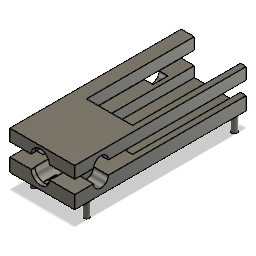
Atari 7800 AV MKII v5 (Autodesk Fusion 360 design; units mm, degrees)
Autodesk Fusion 360 part; units mm, degrees
note: some values were not read from the file. Chosen so that the rebuilt part matches the saved one: which face or edge a step refers to; which pieces of a blend or face edit are solid. Set by a fixed rule: which sketch regions a step uses.
sketch "Sketch1" plane through (0, 0, 0) normal (0, 1, 0) x (1, 0, 0)
  line L0 (0, 0) -> (22, 0)
  line L1 (22, 0) -> (22, -52.5)
  line L2 (22, -52.5) -> (0, -52.5)
  line L3 (0, -52.5) -> (0, 0)
  dimension "d1" = 22
  dimension "d2" = 52.5
  constraint horizontal L0
  constraint vertical L1
  constraint horizontal L2
  constraint vertical L3
  constraint coincident L0.start L3.end
  measures "d1" distance of L0.start L0.end
  measures "d2" distance of L0.start L2.end
extrude "Extrude1" add sketch "Sketch1" along normal blind 2 makes body 1
sketch "Sketch2" plane through (0, 0, 0) normal (0, -1, 0) x (1, 0, 0)
  line L0 (22, 52.5) -> (0, 52.5)
  line L1 (0, 52.5) -> (0, 0)
  line L2 (0, 0) -> (22, 0)
  line L3 (22, 0) -> (22, 52.5)
  line L4 (0, 0) -> (1.35, 0)
  circle A0 centre (1.35, 1) radius 1
  dimension "d5" = 1.35
  dimension "d6" = 2
  constraint coincident L1.end L2.start
  constraint coincident L4.end A0
  measures "d5" distance of L1.end L4.end
  measures "d6" diameter of A0
extrude "Extrude2" add sketch "Sketch2" along normal blind 5 contours A0 bodies 1
sketch "Sketch3" plane through (0, 0, 0) normal (0, 1, 0) x (1, 0, 0)
  line L0 (1.35, 0) -> (17.05, 0)
  circle A0 centre (17.05, -1) radius 1
  point P0 (1.35, 0)
  dimension "d9" = 15.7
  dimension "d10" = 2
  constraint coincident P0 L0.start
  constraint coincident L0.end A0
  measures "d9" distance of P0 L0.end
  measures "d10" diameter of A0
extrude "Extrude3" add sketch "Sketch3" against normal blind 5 bodies 1
sketch "Sketch4" plane through (0, 0, 0) normal (0, 1, 0) x (1, 0, 0)
  line L0 (1.35, -1.9999) -> (1.35, -2.1921)
  line L1 (1.35, -2.1921) -> (1.35, -50.1921)
  circle A0 centre (1.35, -51.1921) radius 1
  point P0 (1.35, 0)
  dimension "d13" = 48
  dimension "d14" = 2
  constraint coincident L1.end A0
  measures "d13" distance of L0.end L1.end
  measures "d14" diameter of A0
extrude "Extrude4" add sketch "Sketch4" against normal blind 5 bodies 1
sketch "Sketch5" plane through (0, 0, 0) normal (0, -1, 0) x (1, 0, 0)
  circle A0 centre (1.35, 51.1921) radius 1
  line L0 (22, 52.5) -> (0, 52.5)
  line L1 (0, 52.5) -> (0, 0)
  line L2 (0, 0) -> (1.35, 0)
  circle A1 centre (1.35, 1) radius 1
  line L3 (1.35, 0) -> (17.05, 0)
  circle A2 centre (17.05, 1) radius 1
  line L4 (17.05, 0) -> (22, 0)
  line L5 (22, 0) -> (22, 52.5)
  line L6 (1.35, 51.1921) -> (1.35, 52.1921)
  line L7 (1.35, 52.1921) -> (17.05, 52.1921)
  circle A3 centre (17.05, 51.1921) radius 1
  dimension "d17" = 15.7
  dimension "d18" = 2
  constraint coincident A0.centre L6.start
  constraint vertical L6
  constraint coincident L7.end A3
  measures "d17" distance of L6.end L7.end
  measures "d18" diameter of A3
extrude "Extrude5" add sketch "Sketch5" along normal blind 5 contours A3 bodies 1
sketch "Sketch6" plane through (0, 0, 52.5) normal (0, 0, 1) x (1, 0, 0)
  line L0 (0, 0) -> (22, 0)
  line L1 (22, 0) -> (22, 2)
  line L2 (22, 2) -> (0, 2)
  line L3 (0, 2) -> (0, 0)
  line L4 (0, 2) -> (13.35, 2)
  line L5 (13.35, 2) -> (13.35, 9)
  circle A0 centre (13.35, 9) radius 3
  dimension "d21" = 13.35
  dimension "d22" = 7
  dimension "d23" = 6
  constraint coincident L2.end L3.start
  constraint coincident L5.end A0.centre
  measures "d21" distance of L2.end L4.end
  measures "d22" distance of L4.end L5.end
  measures "d23" diameter of A0
extrude "Extrude6" add sketch "Sketch6" along normal blind 3 separate body contours A0 makes body 2
sketch "Sketch7" plane through (0, 0, 52.5) normal (0, 0, -1) x (-1, 0, 0)
  circle A0 centre (-13.35, 9) radius 3
  circle A1 centre (-13.35, 9) radius 3.225
  dimension "d26" = 6.45
  constraint concentric A0 A1
  measures "d26" diameter of A1
extrude "Extrude7" add sketch "Sketch7" along normal blind 14.7 contours A0 | A1 bodies 2
sketch "Sketch8" plane through (0, 0, 37.8) normal (0, 0, -1) x (-1, 0, 0)
  circle A0 centre (-13.35, 9) radius 3.225
  circle A1 centre (-13.35, 9) radius 2.725
  dimension "d29" = 5.45
  constraint concentric A0 A1
  measures "d29" diameter of A1
extrude "Extrude8" add sketch "Sketch8" along normal blind 2 and the other way blind -0.5 separate body makes body 3
sketch "Sketch9" plane through (0, 0, 55.5) normal (0, 0, 1) x (1, 0, 0)
  circle A0 centre (13.35, 9) radius 3
  circle A1 centre (13.35, 9) radius 3.075
  circle A2 centre (13.35, 9) radius 3.225
  circle A3 centre (13.35, 9) radius 3.225
  dimension "d34" = 6.15
  constraint concentric A0 A1
  constraint concentric A1 A2
  measures "d34" diameter of A1
extrude "Extrude9" add sketch "Sketch9" along normal blind -2.8 and the other way blind 0.2 separate body contours A2 A3 makes body 4
extrude "Extrude10" add 1 faces at (10.3138, 8.7044, 37.3) along direction (0, 0, 1) blind 0.3 on bodies 3 bodies 3
sketch "Sketch10" plane through (0, 2, 0) normal (0, 1, 0) x (-1, 0, 0)
  line L0 (0, 52.5) -> (-22, 52.5)
  line L1 (-22, 52.5) -> (-22, 0)
  line L2 (-22, 0) -> (0, 0)
  line L3 (0, 0) -> (0, 52.5)
  line L4 (-16.575, 35.8) -> (-10.125, 35.8)
  line L5 (-10.2258, 35.8) -> (1.5, 35.8)
  line L6 (-16.075, 37.6) -> (-26, 37.6)
  line L7 (-22, 37.6) -> (0, 37.6)
  line L8 (0, 37.6) -> (0, 35.8)
  line L9 (0, 35.8) -> (-22, 35.8)
  line L10 (-22, 35.8) -> (-22, 37.6)
  point P0 (-16.075, 37.6)
  constraint coincident L4 L5.start
  constraint perpendicular L3 L5
  constraint coincident P0 L6.start
  constraint parallel L4 L6
  constraint horizontal L7
  constraint vertical L8
  constraint horizontal L9
  constraint vertical L10
  constraint coincident L5 L8.end
  constraint coincident L3 L8.end
  constraint coincident L6 L7.start
  constraint coincident L1 L7.start
extrude "Extrude11" add sketch "Sketch10" along normal blind 4 contours L1 L3 L4 L5 L6 L7 L8 L9 L10 bodies 3 1
sketch "Sketch11" plane through (0, 0, 35.8) normal (0, 0, -1) x (-1, 0, 0)
  arc A0 (-12.1665, 6) -> (-14.5335, 6) centre (-13.35, 9) ccw
  line L0 (-14.5335, 6) -> (-22, 6)
  line L1 (-22, 6) -> (-22, 2)
  line L2 (-22, 2) -> (0, 2)
  line L3 (0, 2) -> (0, 6)
  line L4 (0, 6) -> (-12.1665, 6)
  circle A1 centre (-13.35, 9) radius 2.725
  line L5 (-13.35, 9) -> (-22, 9)
  line L6 (-22, 9) -> (-22, 6)
  line L7 (-13.35, 9) -> (0, 9)
  line L8 (0, 9) -> (0, 6)
  constraint coincident A0.centre A1.centre
  constraint horizontal L5
  constraint coincident L0.end L1.start
  constraint perpendicular L5 L6
  constraint perpendicular L6 L7
  constraint coincident L3.end L4.start
  constraint perpendicular L4 L8
extrude "Extrude12" add sketch "Sketch11" against normal blind 1.8 contours A0 L4 L7 L8 | A0 L0 L5 L6 bodies 3
sketch "Sketch12" plane through (0, 0, 37.6) normal (0, 0, 1) x (1, 0, 0)
  arc A0 (16.575, 9) -> (10.125, 9) centre (13.35, 9) ccw
  line L0 (10.125, 9) -> (0, 9)
  line L1 (0, 9) -> (0, 2)
  line L2 (0, 2) -> (22, 2)
  line L3 (22, 2) -> (22, 9)
  line L4 (22, 9) -> (16.575, 9)
  circle A1 centre (13.35, 9) radius 2.725
  circle A2 centre (13.35, 9) radius 3.25
  dimension "d45" = 6.5
  constraint concentric A0 A2
  measures "d45" diameter of A2
extrude "Extrude13" add sketch "Sketch12" along normal blind 14.5 contours L0 L1 L2 L3 L4 A2 bodies 3
extrude "Extrude14" add 1 faces at (14.6667, 0.6667, 52.5) along direction (0, 0, 1) blind 1 on bodies 3 bodies 3
extrude "Extrude15" add 1 faces at (7.3333, 2, 53.0333) along direction (0, 1, 0) blind 3.8 on bodies 3 bodies 3 4
extrude "Extrude16" add 1 faces at (3.3772, 7.7827, 52.1) along direction (0, 0, 1) blind 1.4 on bodies 3 bodies 3
extrude "Extrude17" add 1 faces at (20.1581, 7.635, 52.1) along direction (0, 0, 1) blind 1.4 on bodies 3 bodies 3
sketch "Sketch13" plane through (22, 0, 0) normal (1, 0, 0) x (0, 0, -1)
  line L0 (-35.8, 2) -> (-35.8, 9)
  line L1 (-35.8, 9) -> (-53.5, 9)
  line L2 (-53.5, 9) -> (-53.5, 0)
  line L3 (-53.5, 0) -> (0, 0)
  line L4 (0, 0) -> (0, 2)
  line L5 (0, 2) -> (-35.8, 2)
  line L6 (-35.8, 9) -> (-56, 9)
  line L7 (-56, 9) -> (-56, 13)
  line L8 (-56, 13) -> (-35.8, 13)
  line L9 (-35.8, 13) -> (-35.8, 9)
  constraint horizontal L6
  constraint vertical L7
  constraint horizontal L8
  constraint vertical L9
  constraint coincident L0.end L1.start
extrude "Extrude18" cut sketch "Sketch13" against normal blind 21 contours L1 L6 L7 L8 L9 bodies 3
extrude "Extrude19" cut 1 faces at (13.2164, 5.8, 52.3) along direction (0, -1, 0) blind 0.1 on bodies 3 bodies 3
extrude "Extrude20" add 1 faces at (12.9492, 5.7667, 52.9667) along direction (1, 0, 0) blind 1.3 on bodies 3 bodies 3
extrude "Extrude21" add 1 faces at (12.9492, 5.7667, 52.9667) along direction (-1, 0, 0) blind 0.69 on bodies 3 bodies 3
extrude "Extrude22" add 1 faces at (12.8935, 5.8, 53.2333) along direction (0, 1, 0) blind 0.05 on bodies 3 bodies 3
extrude "Extrude23" add 1 faces at (13.8065, 5.8, 53.2333) along direction (0, 1, 0) blind 0.06 on bodies 3 bodies 3
move_face "OffsetFaces1" offset 0.6 1 faces at (14.2695, 5.9089, 53.8333) on bodies 3
extrude "Extrude24" cut 1 faces at (16.9108, 8.81, 55.3) along direction (0, 0, -1) blind 1.8 on bodies 3 bodies 3
extrude "Extrude25" add 1 faces at (3.5265, 5.5553, 53.5) along direction (0, 0, 1) blind 0.5 on bodies 3 bodies 3
extrude "Extrude26" add 1 faces at (7.3333, 2, 11.9333) along direction (0, 1, 0) blind 7 on bodies 3 bodies 3
extrude "Extrude27" cut 1 faces at (12.7837, 8.2898, 35.8) along direction (0, 0, -1) blind 36 on bodies 3 bodies 3
sketch "Sketch14" plane through (0, 9, 0) normal (0, 1, 0) x (-1, 0, 0)
  line L0 (-16.075, 0) -> (-16.075, 37.6)
  line L1 (-16.075, 37.6) -> (-16.6, 37.6)
  line L2 (-16.6, 37.6) -> (-16.6, 52.7)
  line L3 (-16.6, 52.7) -> (-16.425, 52.7)
  line L4 (-16.425, 52.7) -> (-16.425, 54)
  line L5 (-16.425, 54) -> (-22, 54)
  line L6 (-22, 54) -> (-22, 0)
  line L7 (-22, 0) -> (-16.075, 0)
  line L8 (-20, 0) -> (-4.4651, 0)
  line L9 (-4.4651, 0) -> (-4.4651, 32.4674)
  line L10 (-4.4651, 32.4674) -> (-20, 32.4674)
  line L11 (-20, 32.4674) -> (-20, 0)
  constraint horizontal L8
  constraint vertical L9
  constraint horizontal L10
  constraint vertical L11
  constraint coincident L7 L8.start
extrude "Extrude28" cut sketch "Sketch14" against normal blind 4 contours L0 L7 L8 L10 L11 | L0 L8 L9 L10 bodies 3
sketch "Sketch15" plane through (0, 0, 54) normal (0, 0, 1) x (1, 0, 0)
  line L0 (10.275, 9) -> (0, 9)
  line L1 (0, 9) -> (0, 0)
  line L2 (0, 0) -> (22, 0)
  line L3 (22, 0) -> (22, 9)
  line L4 (22, 9) -> (16.425, 9)
  arc A0 (10.275, 9) -> (16.425, 9) centre (13.35, 9) ccw
  line L5 (0, 9) -> (22, 9)
  line L6 (22, 9) -> (22, 13)
  line L7 (22, 13) -> (0, 13)
  line L8 (0, 13) -> (0, 9)
  dimension "d79" = 4
  constraint horizontal L5
  constraint vertical L6
  constraint horizontal L7
  constraint vertical L8
  constraint coincident L0.end L1.start
  measures "d79" distance of L0.end L7.end
extrude "Extrude29" add sketch "Sketch15" against normal blind 54 separate body contours L0 L4 L5 L6 L7 L8 makes body 5
sketch "Sketch16" plane through (0, 0, 54) normal (0, 0, 1) x (1, 0, 0)
  line L0 (10.275, 9) -> (0, 9)
  line L1 (0, 9) -> (0, 0)
  line L2 (0, 0) -> (22, 0)
  line L3 (22, 0) -> (22, 9)
  line L4 (22, 9) -> (16.425, 9)
  arc A0 (10.275, 9) -> (16.425, 9) centre (13.35, 9) ccw
  circle A1 centre (13.35, 9) radius 3.075
  constraint concentric A0 A1
extrude "Extrude30" cut sketch "Sketch16" against normal blind 16 contours A0 A1 bodies 5
sketch "Sketch17" plane through (0, 0, 37.6) normal (0, 0, 1) x (1, 0, 0)
  line L0 (10.625, 9) -> (10.1, 9)
  arc A0 (10.1, 9) -> (16.6, 9) centre (13.35, 9) ccw
  line L1 (16.6, 9) -> (16.075, 9)
  arc A1 (10.625, 9) -> (16.075, 9) centre (13.35, 9) ccw
  circle A2 centre (13.35, 9) radius 3.25
  constraint concentric A0 A2
extrude "Extrude31" cut sketch "Sketch17" along normal blind 15.1 bodies 5
sketch "Sketch18" plane through (0, 0, 37.6) normal (0, 0, 1) x (1, 0, 0)
  line L0 (10.625, 9) -> (10.1, 9)
  arc A0 (10.1, 9) -> (16.6, 9) centre (13.35, 9) ccw
  line L1 (16.6, 9) -> (16.075, 9)
  arc A1 (10.625, 9) -> (16.075, 9) centre (13.35, 9) ccw
  circle A2 centre (13.35, 9) radius 2.725
  constraint concentric A0 A2
extrude "Extrude32" cut sketch "Sketch18" against normal blind 40 contours A1 A2 bodies 5
extrude "Extrude33" cut 1 faces at (12.205, 5, 21.6449) along direction (0, 1, 0) blind 10 on bodies 3 bodies 5
extrude "Extrude34" cut 1 faces at (1.6126, -5, 51.6617) along direction (0, 1, 0) blind 5 on bodies 3 bodies 3
extrude "Extrude35" cut 1 faces at (16.7497, -5, 51.3367) along direction (0, 1, 0) blind 5 on bodies 3 bodies 3
extrude "Extrude36" cut 1 faces at (16.476, -5, 0.7236) along direction (0, 1, 0) blind 5 on bodies 3 bodies 3
sketch "Sketch19" plane through (0, 0, 0) normal (0, -1, 0) x (1, 0, 0)
  line L0 (0, 54) -> (0, 0)
  line L1 (0, 0) -> (1.35, 0)
  circle A0 centre (1.35, 1) radius 1
  line L2 (1.35, 0) -> (22, 0)
  line L3 (22, 0) -> (22, 54)
  line L4 (22, 54) -> (0, 54)
  line L5 (0, 54) -> (0, 53)
  circle A1 centre (1, 53) radius 1
  dimension "d96" = 1
  dimension "d97" = 2
  constraint coincident L0.start L4.end
  constraint coincident L5.end A1
  measures "d96" distance of L0.start L5.end
  measures "d97" diameter of A1
extrude "Extrude37" add sketch "Sketch19" along normal blind 5 contours A1 bodies 3
sketch "Sketch20" plane through (0, 0, 0) normal (0, -1, 0) x (1, 0, 0)
  arc A0 (0, 53) -> (1, 54) centre (1, 53) ccw
  line L0 (0, 53) -> (0, 0)
  line L1 (0, 0) -> (1.35, 0)
  circle A1 centre (1.35, 1) radius 1
  line L2 (1.35, 0) -> (22, 0)
  line L3 (22, 0) -> (22, 54)
  line L4 (22, 54) -> (1, 54)
  line L5 (22, 54) -> (22, 53)
  circle A2 centre (21, 53) radius 1
  dimension "d100" = 1
  dimension "d101" = 2
  constraint coincident L3.end L4.start
  constraint coincident L3 L5.end
  constraint perpendicular L4 L5
  constraint coincident L5.end A2
  measures "d100" distance of L3.end L5.end
  measures "d101" diameter of A2
extrude "Extrude38" add sketch "Sketch20" along normal blind 5 contours A2 bodies 3
sketch "Sketch21" plane through (0, 0, 0) normal (0, -1, 0) x (1, 0, 0)
  arc A0 (21, 54) -> (22, 53) centre (21, 53) ccw
  line L0 (21, 54) -> (1, 54)
  arc A1 (0, 53) -> (1, 54) centre (1, 53) ccw
  line L1 (0, 53) -> (0, 0)
  line L2 (0, 0) -> (1.35, 0)
  circle A2 centre (1.35, 1) radius 1
  line L3 (1.35, 0) -> (22, 0)
  line L4 (22, 0) -> (22, 53)
  line L5 (22, 0) -> (21, 0)
  circle A3 centre (21, 1) radius 1
  dimension "d104" = 1
  dimension "d105" = 2
  constraint coincident L3.end L4.start
  constraint coincident L5.end A3
  measures "d104" distance of L3.end L5.end
  measures "d105" diameter of A3
extrude "Extrude39" add sketch "Sketch21" along normal blind 5 contours A3 bodies 3
sketch "Sketch22" plane through (4.4651, 0, 0) normal (1, 0, 0) x (0, 0, -1)
  line L0 (0, 9) -> (-32.4674, 9)
  line L1 (-32.4674, 9) -> (-32.4674, 5)
  line L2 (-32.4674, 5) -> (0, 5)
  line L3 (0, 5) -> (0, 9)
  line L4 (0, 5) -> (-5, 5)
  line L5 (-5, 5) -> (-5, 6)
  line L6 (-5, 6) -> (0, 6)
  line L7 (0, 6) -> (0, 5)
  line L8 (-5, 6) -> (-7.5, 6)
  line L9 (-7.5, 6) -> (-7.5, 5)
  line L10 (-7.5, 5) -> (-5, 5)
  line L11 (-5, 5) -> (-5, 6)
  line L12 (-7.5, 6) -> (-10, 6)
  line L13 (-10, 6) -> (-10, 5)
  line L14 (-10, 5) -> (-7.5, 5)
  line L15 (-7.5, 5) -> (-7.5, 6)
  line L16 (-10, 6) -> (-12.5, 6)
  line L17 (-12.5, 6) -> (-12.5, 5)
  line L18 (-12.5, 5) -> (-10, 5)
  line L19 (-10, 5) -> (-10, 6)
  line L20 (-12.5, 6) -> (-10, 6)
  line L21 (-10, 6) -> (-10, 9)
  line L22 (-10, 9) -> (-12.5, 9)
  line L23 (-12.5, 9) -> (-12.5, 6)
  line L24 (-7.5, 6) -> (-5, 6)
  line L25 (-5, 6) -> (-5, 9)
  line L26 (-5, 9) -> (-7.5, 9)
  line L27 (-7.5, 9) -> (-7.5, 6)
  line L28 (-12.5, 9) -> (-5, 9)
  line L29 (-5, 9) -> (-5, 8)
  line L30 (-5, 8) -> (-12.5, 8)
  line L31 (-12.5, 8) -> (-12.5, 9)
  dimension "d108" = 5
  dimension "d109" = 1
  dimension "d110" = 1
  dimension "d111" = 2.5
  dimension "d112" = 2.5
  dimension "d113" = 1
  dimension "d114" = 2.5
  dimension "d115" = 1
  constraint horizontal L4
  constraint vertical L5
  constraint horizontal L6
  constraint vertical L7
  constraint coincident L2.end L3.start
  constraint horizontal L8
  constraint vertical L9
  constraint horizontal L10
  constraint vertical L11
  constraint horizontal L12
  constraint vertical L13
  constraint horizontal L14
  constraint vertical L15
  constraint horizontal L16
  constraint vertical L17
  constraint horizontal L18
  constraint vertical L19
  constraint horizontal L20
  constraint vertical L21
  constraint horizontal L22
  constraint vertical L23
  constraint coincident L0 L21.end
  constraint horizontal L24
  constraint vertical L25
  constraint horizontal L26
  constraint vertical L27
  constraint coincident L0 L25.end
  constraint horizontal L28
  constraint vertical L29
  constraint horizontal L30
  constraint vertical L31
  constraint coincident L25 L29.end
  measures "d108" distance of L2.end L4.end
  measures "d109" distance of L2.end L6.end
  measures "d110" distance of L5.end L4.end
  measures "d111" distance of L5.end L8.end
  measures "d112" distance of L8.end L12.end
  measures "d113" distance of L8.end L9.end
  measures "d114" distance of L12.end L16.end
  measures "d115" distance of L12.end L13.end
extrude "Extrude40" add sketch "Sketch22" along normal blind 17 contours L0 L25 L26 L27 L28 L29 L30 | L0 L21 L22 L23 L28 L30 L31 bodies 3
extrude "Extrude41" cut 1 faces at (1.2554, -5, 53.3747) along direction (0, 1, 0) blind 5 on bodies 3 bodies 3
extrude "Extrude42" cut 1 faces at (1.0981, -5, 1.5651) along direction (0, 1, 0) blind 5 on bodies 3 bodies 3
extrude "Extrude43" cut 1 faces at (20.5597, -5, 0.788) along direction (0, 1, 0) blind 5 on bodies 3 bodies 3
sketch "Sketch23" plane through (0, 0, 0) normal (0, -1, 0) x (1, 0, 0)
  line L0 (21, 54) -> (0, 54)
  line L1 (0, 54) -> (0, 0)
  line L2 (0, 0) -> (22, 0)
  line L3 (22, 0) -> (22, 53)
  arc A0 (21, 54) -> (22, 53) centre (21, 53) ccw
  circle A1 centre (21, 3) radius 1
  circle A2 centre (3.35, 3) radius 1
  circle A3 centre (3.35, 53) radius 1
  dimension "d124" = 50
  dimension "d125" = 2
  dimension "d126" = 17.65
  dimension "d127" = 2
  dimension "d128" = 50
  dimension "d129" = 2
  measures "d124" distance of A0.centre A1.centre
  measures "d125" diameter of A1
  measures "d126" distance of A1.centre A2.centre
  measures "d127" diameter of A2
  measures "d128" distance of A2.centre A3.centre
  measures "d129" diameter of A3
extrude "Extrude44" add sketch "Sketch23" along normal blind 5 contours A3 | A1 | A2 bodies 3
move_face "MoveFace1" to x (1, 0, 0) y (0, 1, 0) z (0, 0, 1) at (-3, 0, 0) 11 faces at (13.2733, 5.926, 53.6667) (13.4267, 5.926, 53.2333) (13.2734, 5.7779, 52.7) (11.523, 6.3122, 42.6333) (16.4028, 8.7032, 37.6) (10.6385, 8.7287, 37) (10.6385, 8.7287, 34.6891) (12.7821, 5.7333, 52.5) (13.5393, 5.7, 52.3) (13.9179, 5.7333, 52.5) (13.792, 5.7519, 52.1) on bodies 3
move_face "MoveFace2" to x (1, 0, 0) y (0, 1, 0) z (0, 0, 1) at (-3, 0, 0) 5 faces at (11.3153, 11.3056, 53.5667) (16.596, 9.162, 42.6333) (16.4028, 9.2968, 37.6) (15.9907, 9.6724, 34.1783) (16.5181, 9.3142, 52.7) on bodies 5
sketch "Sketch24" plane through (0, 0, 0) normal (-1, 0, 0) x (0, 0, 1)
  line L0 (54, 9) -> (0, 9)
  line L1 (0, 9) -> (0, 0)
  line L2 (0, 0) -> (54, 0)
  line L3 (54, 0) -> (54, 9)
  circle A0 centre (10, 9) radius 2.5
  circle A1 centre (45.15, 9) radius 2.5
  line L4 (52.7, 9) -> (37.6, 9)
  point P0 (10, 9)
  dimension "d132" = 5
  dimension "d133" = 5
  constraint coincident P0 A0.centre
  constraint midpoint A1.centre L4
  measures "d132" diameter of A0
  measures "d133" diameter of A1
extrude "Extrude45" cut sketch "Sketch24" against normal blind 3 contours L0 A1 L4 | L0 A1 L4 | L0 A0 | L0 A0 bodies 3 5
sketch "Sketch25" plane through (22, 0, 0) normal (1, 0, 0) x (0, 0, -1)
  line L0 (0, 9) -> (-54, 9)
  line L1 (-54, 9) -> (-54, 0)
  line L2 (-54, 0) -> (-53, 0)
  line L3 (-53, 0) -> (-3, 0)
  line L4 (-3, 0) -> (0, 0)
  line L5 (0, 0) -> (0, 9)
  circle A0 centre (-45.15, 9) radius 2.5
  line L6 (-47.65, 9) -> (-42.65, 9)
  dimension "d136" = 5
  constraint midpoint A0.centre L6
  measures "d136" diameter of A0
extrude "Extrude46" cut sketch "Sketch25" against normal blind 5 contours L0 A0 L6 | L0 A0 L6 bodies 3 5
extrude "Extrude47" cut 2 faces at (3, 9.3616, 45.9008) (3, 8.3928, 44.3622) along direction (1, 0, 0) blind 2 on bodies 3 5 bodies 3 5
move_face "MoveFace3" to x (1, 0, 0) y (0, 1, 0) z (0, 0, 1) at (0, 0, 4) 11 faces at (18.7068, 5.5553, 54) (12.3847, 6.6944, 53.1333) (18.6667, 8.8754, 42.6531) (2, 8.8754, 47.6469) (4.3333, 8.8754, 47.6469) (5, 8.3928, 44.3622) (17, 8.3928, 45.9378) (10.4266, 5.7779, 52.7) (13.4028, 8.7032, 37.6) (7.6385, 8.7287, 35.8891) (17.6513, 7.3989, 32.4674) on bodies 3
extrude "Extrude48" add 1 faces at (9.6434, 8.6667, 12.5) along direction (0, 0, 1) blind 7 on bodies 3 bodies 3
extrude "Extrude49" cut 1 faces at (9.6434, 8.3333, 10) along direction (0, 0, 1) blind 7 on bodies 3 bodies 3
extrude "Extrude50" add 1 faces at (9.6434, 8.6667, 7.5) along direction (0, 0, 1) blind 5 on bodies 3 bodies 3
extrude "Extrude51" cut 1 faces at (9.6434, 8.6667, 5) along direction (0, 0, 1) blind 5 on bodies 3 bodies 3
move_face "MoveFace4" to x (1, 0, 0) y (0, 1, 0) z (0, 0, 1) at (0, 0, 4) 9 faces at (19.0961, 10.6355, 54) (1.6667, 9.2489, 42.6624) (17.5333, 9, 51.45) (8.3153, 11.3056, 53.5667) (5, 9.3616, 45.9008) (8.6787, 11.5718, 37.6) (11.6619, 11.9008, 52.7) (18.6667, 9.8551, 47.4992) (17, 9.3616, 44.3992) on bodies 5
move_face "MoveFace5" by (0, 0, 4) 1 faces at (17.6513, 10.6011, 32.4674) on bodies 5
move_face "MoveFace6" to x (1, 0, 0) y (0, 1, 0) z (0, 0, 1) at (0, -4.5, 0) 11 faces at (10.5393, 5.7, 53.6333) (11.2739, 5.8841, 49.6) (7.679, 8.4601, 38.1783) (1.4884, 9, 31.8725) (1.6667, 6.5934, 49.8271) (2, 8.8754, 12.4969) (9.6434, 8.6667, 19.5) (14.8217, 5, 24.3116) (9.6434, 8.6667, 12.5) (18.6667, 6.8999, 50.5064) (8.9472, 6.2636, 57.5667) on bodies 3
move_face "MoveFace7" by (0, 0.5, 0) 1 faces at (9.6434, 0.5, 12.1558) on bodies 3
hidden bodies 2
